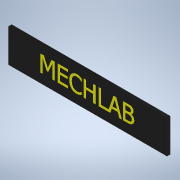
# Autodesk Inventor part: Arcade_TopName
Saved by Autodesk Inventor 2022 (Build 260153000, 153)
## iProperties
Created: 2023-12-22
Part Number: Arcade_TopName
Material: Generic
Document SubType Name: Modeling
Designer: Petr Černý
Density: 1 g/cm^3
Appearance: Default
Author: Petr Černý
Autodesk Inventor part; units mm, degrees
ref_plane "YZ Plane" through (0, 0, 0) normal (1, 0, 0) x (0, 1, 0)
ref_plane "XZ Plane" through (0, 0, 0) normal (0, 1, 0) x (-1, 0, 0)
ref_plane "XY Plane" through (0, 0, 0) normal (0, 0, 1) x (1, 0, 0)
sketch "Sketch1" plane through (0, 0, 0) normal (0, 0, 1) x (1, 0, 0)
  line L0 (-19.2992, 6.7536) -> (470.7008, 6.7536)
  line L1 (470.7008, 6.7536) -> (470.7008, -96.2464)
  line L2 (470.7008, -96.2464) -> (-19.2992, -96.2464)
  line L3 (-19.2992, -96.2464) -> (-19.2992, 6.7536)
  point P0 (0, 0)
  dimension "d0" = 490
  dimension "d1" = 103
  constraints: 8 end point, 2 parallel, 1 horizontal, 1 perpendicular
  measures "d0" distance of L1.end L2.end
  measures "d1" distance of L0.end L1.end
extrude "Extrusion1" add sketch "Sketch1" along normal blind 15
sketch "Sketch2" plane through (470.7008, -96.2464, 0) normal (1, 0, 0) x (0, 0, -1)
  line L0 (0, 103) -> (-15, 103) projected
  line L1 (0, 103) -> (-5, 103)
  line L2 (-5, 103) -> (-5, 0)
  line L3 (-5, 0) -> (0, 0)
  line L4 (0, 0) -> (0, 103)
  point P0 (0, 96.2464)
  dimension "d4" = 5
  dimension "d5" = 103
  constraints: 8 end point, 2 parallel, 1 horizontal, 1 perpendicular
  measures "d4" distance of L3.end L2.end
  measures "d5" distance of L2.end L1.end
extrude "Extrusion2" cut sketch "Sketch2" against normal blind 7
sketch "Sketch3" plane through (-19.2992, -96.2464, 0) normal (-1, 0, 0) x (0, 0, 1)
  line L0 (5, 0) -> (5, 103) projected
  line L1 (0, 103) -> (5, 103)
  line L2 (5, 103) -> (5, 0)
  line L3 (5, 0) -> (0, 0)
  line L4 (0, 0) -> (0, 103)
  point P0 (0, 96.2464)
  dimension "d8" = 5
  dimension "d9" = 103
  constraints: 8 end point, 2 parallel, 1 horizontal, 1 perpendicular
  measures "d8" distance of L0.start L3.end
  measures "d9" distance of L1.end L0.start
extrude "Extrusion3" cut sketch "Sketch3" against normal blind 7
sketch "Sketch4" plane through (-19.2992, 6.7536, 15) normal (0, 1, 0) x (1, 0, 0)
  line L0 (7, 10) -> (7, 15) projected
  line L1 (483, 10) -> (483, 15) projected
  line L2 (7, 15) -> (483, 15)
  line L3 (483, 15) -> (483, 10)
  line L4 (483, 10) -> (7, 10)
  line L5 (7, 10) -> (7, 15)
  point P0 (19.2992, 15)
  constraints: 8 end point, 2 parallel, 1 horizontal, 1 perpendicular
extrude "Extrusion4" cut sketch "Sketch4" against normal blind 15
sketch "Sketch5" plane through (0, 0, 15) normal (0, 0, 1) x (1, 0, 0)
  line L0 (75.7008, -15.9052) -> (425.7008, -15.9052) construction
  line L1 (425.7008, -15.9052) -> (425.7008, -75.4937) construction
  line L2 (425.7008, -75.4937) -> (75.7008, -75.4937) construction
  line L3 (75.7008, -75.4937) -> (75.7008, -15.9052) construction
  line L4 (-19.2992, 6.7536) -> (-19.2992, -96.2464) projected
  line L5 (470.7008, -96.2464) -> (470.7008, 6.7536) projected
  line L6 (123.6344, -66.7966) -> (116.9893, -66.7966)
  line L7 (116.9893, -66.7966) -> (116.9893, -23.7253)
  line L8 (116.9893, -23.7253) -> (103.9423, -53.0203)
  line L9 (103.9423, -53.0203) -> (99.8904, -53.0203)
  line L10 (99.8904, -53.0203) -> (86.965, -23.7253)
  line L11 (86.965, -23.7253) -> (86.965, -66.7966)
  line L12 (86.965, -66.7966) -> (80.7656, -66.7966)
  line L13 (80.7656, -66.7966) -> (80.7656, -16.7966)
  line L14 (80.7656, -16.7966) -> (89.8418, -16.7966)
  line L15 (89.8418, -16.7966) -> (102.3216, -44.6329)
  line L16 (102.3216, -44.6329) -> (114.3961, -16.7966)
  line L17 (114.3961, -16.7966) -> (123.6344, -16.7966)
  line L18 (123.6344, -16.7966) -> (123.6344, -66.7966)
  line L19 (133.764, -66.7966) -> (133.764, -16.7966)
  line L20 (133.764, -16.7966) -> (165.0444, -16.7966)
  line L21 (165.0444, -16.7966) -> (165.0444, -22.7123)
  line L22 (165.0444, -22.7123) -> (140.4091, -22.7123)
  line L23 (140.4091, -22.7123) -> (140.4091, -36.4076)
  line L24 (140.4091, -36.4076) -> (163.3831, -36.4076)
  line L25 (163.3831, -36.4076) -> (163.3831, -42.3234)
  line L26 (163.3831, -42.3234) -> (140.4091, -42.3234)
  line L27 (140.4091, -42.3234) -> (140.4091, -60.8809)
  line L28 (140.4091, -60.8809) -> (165.0444, -60.8809)
  line L29 (165.0444, -60.8809) -> (165.0444, -66.7966)
  line L30 (165.0444, -66.7966) -> (133.764, -66.7966)
  spline S0 degree 2 poles (191.8677, -67.688) (187.0055, -67.688) (178.7802, -64.406) (175.7818, -61.124) knots 0 0 0 1 2 2 2
  spline S1 degree 2 poles (175.7818, -61.124) (172.7835, -57.8825) (169.5015, -48.158) (169.5015, -41.8371) knots 0 0 0 1 2 2 2
  spline S2 degree 2 poles (169.5015, -41.8371) (169.5015, -35.5568) (172.7024, -26.2375) (175.7413, -22.7934) knots 0 0 0 1 2 2 2
  spline S3 degree 2 poles (175.7413, -22.7934) (178.7397, -19.4303) (186.9245, -15.9052) (191.9893, -15.9052) knots 0 0 0 1 2 2 2
  spline S4 degree 2 poles (191.9893, -15.9052) (194.5015, -15.9052) (198.918, -16.6345) (200.7818, -17.2018) knots 0 0 0 1 2 2 2
  spline S5 degree 2 poles (200.7818, -17.2018) (202.4026, -17.7285) (205.7656, -19.2277) (207.4269, -20.1191) knots 0 0 0 1 2 2 2
  line L31 (207.4269, -20.1191) -> (207.4269, -28.1418)
  line L32 (207.4269, -28.1418) -> (206.9002, -28.1418)
  spline S6 degree 2 poles (206.9002, -28.1418) (206.0087, -27.3315) (203.2535, -25.0624) (201.2681, -23.9684) knots 0 0 0 1 2 2 2
  spline S7 degree 2 poles (201.2681, -23.9684) (199.3637, -22.9149) (194.8661, -21.5778) (191.9488, -21.5778) knots 0 0 0 1 2 2 2
  spline S8 degree 2 poles (191.9488, -21.5778) (188.7478, -21.5778) (183.0347, -24.2115) (180.8872, -26.7237) knots 0 0 0 1 2 2 2
  spline S9 degree 2 poles (180.8872, -26.7237) (178.7802, -29.2764) (176.4301, -37.0154) (176.4301, -41.8371) knots 0 0 0 1 2 2 2
  spline S10 degree 2 poles (176.4301, -41.8371) (176.4301, -46.983) (178.9018, -54.3979) (181.0493, -56.9506) knots 0 0 0 1 2 2 2
  spline S11 degree 2 poles (181.0493, -56.9506) (183.1562, -59.4222) (188.7883, -61.9344) (191.9488, -61.9344) knots 0 0 0 1 2 2 2
  spline S12 degree 2 poles (191.9488, -61.9344) (194.8256, -61.9344) (199.7284, -60.5162) (201.6327, -59.4627) knots 0 0 0 1 2 2 2
  spline S13 degree 2 poles (201.6327, -59.4627) (203.4561, -58.4093) (206.1708, -56.2213) (206.9407, -55.4514) knots 0 0 0 1 2 2 2
  line L33 (206.9407, -55.4514) -> (207.4269, -55.4514)
  line L34 (207.4269, -55.4514) -> (207.4269, -63.3931)
  spline S14 degree 2 poles (207.4269, -63.3931) (205.7656, -64.1629) (202.8483, -65.5811) (200.7818, -66.2294) knots 0 0 0 1 2 2 2
  spline S15 degree 2 poles (200.7818, -66.2294) (198.5938, -66.9587) (194.8661, -67.688) (191.8677, -67.688) knots 0 0 0 1 2 2 2
  line L35 (249.931, -66.7966) -> (243.2859, -66.7966)
  line L36 (243.2859, -66.7966) -> (243.2859, -42.3234)
  line L37 (243.2859, -42.3234) -> (220.2713, -42.3234)
  line L38 (220.2713, -42.3234) -> (220.2713, -66.7966)
  line L39 (220.2713, -66.7966) -> (213.6263, -66.7966)
  line L40 (213.6263, -66.7966) -> (213.6263, -16.7966)
  line L41 (213.6263, -16.7966) -> (220.2713, -16.7966)
  line L42 (220.2713, -16.7966) -> (220.2713, -36.4076)
  line L43 (220.2713, -36.4076) -> (243.2859, -36.4076)
  line L44 (243.2859, -36.4076) -> (243.2859, -16.7966)
  line L45 (243.2859, -16.7966) -> (249.931, -16.7966)
  line L46 (249.931, -16.7966) -> (249.931, -66.7966)
  line L47 (289.0314, -66.7966) -> (260.0606, -66.7966)
  line L48 (260.0606, -66.7966) -> (260.0606, -16.7966)
  line L49 (260.0606, -16.7966) -> (266.7057, -16.7966)
  line L50 (266.7057, -16.7966) -> (266.7057, -60.8809)
  line L51 (266.7057, -60.8809) -> (289.0314, -60.8809)
  line L52 (289.0314, -60.8809) -> (289.0314, -66.7966)
  line L53 (288.8694, -66.7966) -> (305.7251, -16.7966)
  line L54 (305.7251, -16.7966) -> (313.9099, -16.7966)
  line L55 (313.9099, -16.7966) -> (330.7656, -66.7966)
  line L56 (330.7656, -66.7966) -> (323.7559, -66.7966)
  line L57 (323.7559, -66.7966) -> (319.2178, -52.8177)
  line L58 (319.2178, -52.8177) -> (300.1335, -52.8177)
  line L59 (300.1335, -52.8177) -> (295.5955, -66.7966)
  line L60 (295.5955, -66.7966) -> (288.8694, -66.7966)
  line L61 (317.3945, -47.1451) -> (309.6554, -23.6038)
  line L62 (309.6554, -23.6038) -> (301.9569, -47.1451)
  line L63 (301.9569, -47.1451) -> (317.3945, -47.1451)
  spline S16 degree 2 poles (369.4204, -51.4401) (369.4204, -55.1678) (366.5841, -60.8809) (364.234, -62.7448) knots 0 0 0 1 2 2 2
  spline S17 degree 2 poles (364.234, -62.7448) (361.3977, -64.9328) (354.9553, -66.7966) (349.8499, -66.7966) knots 0 0 0 1 2 2 2
  line L64 (349.8499, -66.7966) -> (335.5063, -66.7966)
  line L65 (335.5063, -66.7966) -> (335.5063, -16.7966)
  line L66 (335.5063, -16.7966) -> (348.7559, -16.7966)
  spline S18 degree 2 poles (348.7559, -16.7966) (354.1044, -16.7966) (359.4528, -17.4854) (361.884, -18.8226) knots 0 0 0 1 2 2 2
  spline S19 degree 2 poles (361.884, -18.8226) (364.5987, -20.2407) (367.0703, -24.9003) (367.0703, -28.0608) knots 0 0 0 1 2 2 2
  spline S20 degree 2 poles (367.0703, -28.0608) (367.0703, -31.5859) (363.3426, -37.1775) (360.0606, -38.7577) knots 0 0 0 1 2 2 2
  line L67 (360.0606, -38.7577) -> (360.0606, -39.0008)
  spline S21 degree 2 poles (360.0606, -39.0008) (364.5177, -40.2164) (369.4204, -46.6589) (369.4204, -51.4401) knots 0 0 0 1 2 2 2
  spline S22 degree 2 poles (362.4917, -51.7237) (362.4917, -48.8874) (360.871, -45.2407) (358.4399, -43.9441) knots 0 0 0 1 2 2 2
  spline S23 degree 2 poles (358.4399, -43.9441) (356.8596, -43.1337) (353.1319, -42.6475) (349.6878, -42.6475) knots 0 0 0 1 2 2 2
  line L68 (349.6878, -42.6475) -> (342.1514, -42.6475)
  line L69 (342.1514, -42.6475) -> (342.1514, -61.124)
  line L70 (342.1514, -61.124) -> (347.5404, -61.124)
  spline S24 degree 2 poles (347.5404, -61.124) (351.9164, -61.124) (356.9407, -60.3136) (358.8856, -59.017) knots 0 0 0 1 2 2 2
  spline S25 degree 2 poles (358.8856, -59.017) (360.7494, -57.6799) (362.4917, -54.3574) (362.4917, -51.7237) knots 0 0 0 1 2 2 2
  spline S26 degree 2 poles (360.1417, -28.9927) (360.1417, -27.2099) (358.9261, -24.5357) (357.589, -23.7658) knots 0 0 0 1 2 2 2
  spline S27 degree 2 poles (357.589, -23.7658) (355.9682, -22.8744) (352.0379, -22.4692) (348.5128, -22.4692) knots 0 0 0 1 2 2 2
  line L71 (348.5128, -22.4692) -> (342.1514, -22.4692)
  line L72 (342.1514, -22.4692) -> (342.1514, -37.0965)
  line L73 (342.1514, -37.0965) -> (349.6878, -37.0965)
  spline S28 degree 2 poles (349.6878, -37.0965) (352.8078, -37.0965) (355.7656, -36.4482) (357.3459, -35.4352) knots 0 0 0 1 2 2 2
  spline S29 degree 2 poles (357.3459, -35.4352) (358.8856, -34.4627) (360.1417, -31.3428) (360.1417, -28.9927) knots 0 0 0 1 2 2 2
  point P0 (0, 0)
  dimension "d14" = 95
  constraints: 2 other
  measures "d14" distance between parallel lines of L4 L3
emboss "Emboss1" sketch "Sketch5" operation add depth 1 direction (0, 0, -1)
body "Solid1"
